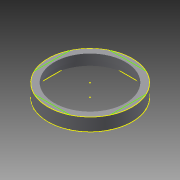
# Autodesk Inventor part: I53O
Saved by Autodesk Inventor 2014 (Build 180170000, 170)
## iProperties
Created: 2013-05-25
Part Number: I53O
Material: Generisch
Document SubType Name: Modeling
Designer: Felix
Density: 1 g/cm^3
Appearance: Vorgabe
Author: Felix
Autodesk Inventor part; units mm, degrees
ref_plane "YZ Plane" through (0, 0, 0) normal (1, 0, 0) x (0, 1, 0)
ref_plane "XZ Plane" through (0, 0, 0) normal (0, 1, 0) x (-1, 0, 0)
ref_plane "XY Plane" through (0, 0, 0) normal (0, 0, 1) x (1, 0, 0)
sketch "Sketch1" plane through (0, 0, 0) normal (0, 0, 1) x (1, 0, 0)
  circle A0 centre (0, 0) radius 13.0482
  spline S0 degree 3 poles (1.4215, 11.0572) (1.4473, 10.9809) (1.4859, 10.8664) (1.5292, 10.7112) (1.5586, 10.5939) (1.5843, 10.4759) (1.6059, 10.357) (1.6236, 10.2374) (1.631, 10.1572) (1.6346, 10.117) knots -0.096663 -0.096663 -0.096663 -0.096663 -0.072499 -0.060415 -0.048332 -0.036249 -0.024166 -0.012083 0 0 0 0 projected
  arc A1 (1.9905, 10.0531) -> (1.6346, 10.117) centre (0, 0) ccw projected
  spline S1 degree 3 poles (1.9905, 10.0531) (2.0079, 10.0894) (2.0426, 10.1621) (2.1009, 10.268) (2.1626, 10.3719) (2.2278, 10.4737) (2.2962, 10.5733) (2.3908, 10.7038) (2.4669, 10.7977) (2.5176, 10.8602) knots -0.096663 -0.096663 -0.096663 -0.096663 -0.084581 -0.072498 -0.060415 -0.048331 -0.036248 -0.024165 0 0 0 0 projected
  arc A2 (2.7193, 10.8115) -> (2.5176, 10.8602) centre (0, 0) ccw projected
  spline S2 degree 3 poles (2.7193, 10.8115) (2.7359, 10.7327) (2.7607, 10.6144) (2.7853, 10.4551) (2.8006, 10.3353) (2.8122, 10.215) (2.8196, 10.0943) (2.8231, 9.9735) (2.8208, 9.893) (2.8197, 9.8527) knots -0.096663 -0.096663 -0.096663 -0.096663 -0.072499 -0.060415 -0.048332 -0.036249 -0.024166 -0.012083 0 0 0 0 projected
  arc A3 (3.1655, 9.7471) -> (2.8197, 9.8527) centre (0, 0) ccw projected
  spline S3 degree 3 poles (3.1655, 9.7471) (3.1871, 9.7811) (3.2302, 9.8492) (3.3006, 9.9475) (3.3741, 10.0433) (3.4509, 10.1367) (3.5306, 10.2275) (3.64, 10.3459) (3.7266, 10.4301) (3.7844, 10.4863) knots -0.096663 -0.096663 -0.096663 -0.096663 -0.084581 -0.072498 -0.060415 -0.048331 -0.036248 -0.024165 0 0 0 0 projected
  arc A4 (3.9789, 10.414) -> (3.7844, 10.4863) centre (0, 0) ccw projected
  spline S4 degree 3 poles (3.9789, 10.414) (3.986, 10.3337) (3.9967, 10.2134) (4.0023, 10.0523) (4.0033, 9.9315) (4.0006, 9.8106) (3.9937, 9.69) (3.9828, 9.5696) (3.9711, 9.4899) (3.9652, 9.45) knots -0.096663 -0.096663 -0.096663 -0.096663 -0.072499 -0.060415 -0.048332 -0.036249 -0.024166 -0.012083 0 0 0 0 projected
  arc A5 (4.2961, 9.3043) -> (3.9652, 9.45) centre (0, 0) ccw projected
  spline S5 degree 3 poles (4.2961, 9.3043) (4.3215, 9.3355) (4.3724, 9.398) (4.4539, 9.4873) (4.5383, 9.5738) (4.6256, 9.6574) (4.7154, 9.7382) (4.838, 9.8428) (4.9341, 9.9161) (4.9981, 9.9651) knots -0.096663 -0.096663 -0.096663 -0.096663 -0.084581 -0.072498 -0.060415 -0.048331 -0.036248 -0.024165 0 0 0 0 projected
  arc A6 (5.1827, 9.8703) -> (4.9981, 9.9651) centre (0, 0) ccw projected
  spline S6 degree 3 poles (5.1827, 9.8703) (5.1803, 9.7898) (5.1766, 9.669) (5.1631, 9.5084) (5.1498, 9.3883) (5.1328, 9.2686) (5.1117, 9.1496) (5.0867, 9.0314) (5.0656, 8.9536) (5.0551, 8.9147) knots -0.096663 -0.096663 -0.096663 -0.096663 -0.072499 -0.060415 -0.048332 -0.036249 -0.024166 -0.012083 0 0 0 0 projected
  arc A7 (5.3664, 8.7309) -> (5.0551, 8.9147) centre (0, 0) ccw projected
  spline S7 degree 3 poles (5.3664, 8.7309) (5.3954, 8.7589) (5.4533, 8.8149) (5.5447, 8.8939) (5.6388, 8.9698) (5.7353, 9.0425) (5.8341, 9.1121) (5.9682, 9.2015) (6.0723, 9.263) (6.1416, 9.304) knots -0.096663 -0.096663 -0.096663 -0.096663 -0.084581 -0.072498 -0.060415 -0.048331 -0.036248 -0.024165 0 0 0 0 projected
  arc A8 (6.3137, 9.1881) -> (6.1416, 9.304) centre (0, 0) ccw projected
  spline S8 degree 3 poles (6.3137, 9.1881) (6.3018, 9.1084) (6.2839, 8.9889) (6.2515, 8.831) (6.2241, 8.7133) (6.193, 8.5965) (6.158, 8.4808) (6.1192, 8.3664) (6.089, 8.2916) (6.074, 8.2543) knots -0.096663 -0.096663 -0.096663 -0.096663 -0.072499 -0.060415 -0.048332 -0.036249 -0.024166 -0.012083 0 0 0 0 projected
  arc A9 (6.3614, 8.0349) -> (6.074, 8.2543) centre (0, 0) ccw projected
  spline S9 degree 3 poles (6.3614, 8.0349) (6.3934, 8.0593) (6.4576, 8.108) (6.5577, 8.1757) (6.6601, 8.24) (6.7646, 8.3007) (6.8709, 8.3581) (7.0146, 8.431) (7.1252, 8.4798) (7.1989, 8.5123) knots -0.096663 -0.096663 -0.096663 -0.096663 -0.084581 -0.072498 -0.060415 -0.048331 -0.036248 -0.024165 0 0 0 0 projected
  arc A10 (7.3561, 8.3768) -> (7.1989, 8.5123) centre (0, 0) ccw projected
  spline S10 degree 3 poles (7.3561, 8.3768) (7.3348, 8.2991) (7.3029, 8.1825) (7.2521, 8.0296) (7.2109, 7.916) (7.1663, 7.8037) (7.1179, 7.693) (7.0657, 7.5839) (7.027, 7.5133) (7.0076, 7.478) knots -0.096663 -0.096663 -0.096663 -0.096663 -0.072499 -0.060415 -0.048332 -0.036249 -0.024166 -0.012083 0 0 0 0 projected
  arc A11 (7.267, 7.2261) -> (7.0076, 7.478) centre (0, 0) ccw projected
  spline S11 degree 3 poles (7.267, 7.2261) (7.3017, 7.2465) (7.3712, 7.2874) (7.4787, 7.3427) (7.5879, 7.3944) (7.6988, 7.4424) (7.8112, 7.4868) (7.9625, 7.5422) (8.0781, 7.5775) (8.1552, 7.6011) knots -0.096663 -0.096663 -0.096663 -0.096663 -0.084581 -0.072498 -0.060415 -0.048331 -0.036248 -0.024165 0 0 0 0 projected
  arc A12 (8.2952, 7.448) -> (8.1552, 7.6011) centre (0, 0) ccw projected
  spline S12 degree 3 poles (8.2952, 7.448) (8.2649, 7.3734) (8.2194, 7.2614) (8.1509, 7.1155) (8.0966, 7.0076) (8.039, 6.9013) (7.9778, 6.7971) (7.9131, 6.695) (7.8663, 6.6294) (7.8429, 6.5967) knots -0.096663 -0.096663 -0.096663 -0.096663 -0.072499 -0.060415 -0.048332 -0.036249 -0.024166 -0.012083 0 0 0 0 projected
  arc A13 (8.0707, 6.3159) -> (7.8429, 6.5967) centre (0, 0) ccw projected
  spline S13 degree 3 poles (8.0707, 6.3159) (8.1076, 6.3321) (8.1814, 6.3644) (8.2946, 6.4066) (8.4092, 6.4451) (8.525, 6.4796) (8.6419, 6.5104) (8.7987, 6.5475) (8.9176, 6.5689) (8.9969, 6.5832) knots -0.096663 -0.096663 -0.096663 -0.096663 -0.084581 -0.072498 -0.060415 -0.048331 -0.036248 -0.024165 0 0 0 0 projected
  arc A14 (9.1179, 6.4146) -> (8.9969, 6.5832) centre (0, 0) ccw projected
  spline S14 degree 3 poles (9.1179, 6.4146) (9.079, 6.3441) (9.0206, 6.2383) (8.9352, 6.1016) (8.8686, 6.0008) (8.7988, 5.9021) (8.7257, 5.8059) (8.6494, 5.7121) (8.5952, 5.6525) (8.568, 5.6228) knots -0.096663 -0.096663 -0.096663 -0.096663 -0.072499 -0.060415 -0.048332 -0.036249 -0.024166 -0.012083 0 0 0 0 projected
  arc A15 (8.761, 5.317) -> (8.568, 5.6228) centre (0, 0) ccw projected
  spline S15 degree 3 poles (8.761, 5.317) (8.7996, 5.3287) (8.8767, 5.3521) (8.9941, 5.3806) (9.1125, 5.4052) (9.2316, 5.4258) (9.3512, 5.4426) (9.5113, 5.4609) (9.632, 5.4681) (9.7124, 5.4729) knots -0.096663 -0.096663 -0.096663 -0.096663 -0.084581 -0.072498 -0.060415 -0.048331 -0.036248 -0.024165 0 0 0 0 projected
  arc A16 (9.8126, 5.2912) -> (9.7124, 5.4729) centre (0, 0) ccw projected
  spline S16 degree 3 poles (9.8126, 5.2912) (9.7656, 5.2258) (9.6951, 5.1276) (9.5942, 5.002) (9.516, 4.9097) (9.4351, 4.82) (9.3511, 4.7331) (9.2643, 4.649) (9.2034, 4.5963) (9.1729, 4.5699) knots -0.096663 -0.096663 -0.096663 -0.096663 -0.072499 -0.060415 -0.048332 -0.036249 -0.024166 -0.012083 0 0 0 0 projected
  arc A17 (9.3284, 4.2435) -> (9.1729, 4.5699) centre (0, 0) ccw projected
  spline S17 degree 3 poles (9.3284, 4.2435) (9.3681, 4.2506) (9.4474, 4.2647) (9.5674, 4.2791) (9.6878, 4.2896) (9.8085, 4.2959) (9.9293, 4.2984) (10.0904, 4.2976) (10.2111, 4.2905) (10.2915, 4.2858) knots -0.096663 -0.096663 -0.096663 -0.096663 -0.084581 -0.072498 -0.060415 -0.048331 -0.036248 -0.024165 0 0 0 0 projected
  arc A18 (10.3695, 4.0935) -> (10.2915, 4.2858) centre (0, 0) ccw projected
  spline S18 degree 3 poles (10.3695, 4.0935) (10.3151, 4.0341) (10.2335, 3.9449) (10.1184, 3.8321) (10.0299, 3.7498) (9.939, 3.6703) (9.8453, 3.5939) (9.7491, 3.5206) (9.6824, 3.4755) (9.649, 3.4529) knots -0.096663 -0.096663 -0.096663 -0.096663 -0.072499 -0.060415 -0.048332 -0.036249 -0.024166 -0.012083 0 0 0 0 projected
  arc A19 (9.7648, 3.1104) -> (9.649, 3.4529) centre (0, 0) ccw projected
  spline S19 degree 3 poles (9.7648, 3.1104) (9.805, 3.1127) (9.8855, 3.1174) (10.0063, 3.1175) (10.1271, 3.1136) (10.2477, 3.1056) (10.368, 3.0939) (10.5279, 3.074) (10.6469, 3.0527) (10.7262, 3.0385) knots -0.096663 -0.096663 -0.096663 -0.096663 -0.084581 -0.072498 -0.060415 -0.048331 -0.036248 -0.024165 0 0 0 0 projected
  arc A20 (10.7809, 2.8383) -> (10.7262, 3.0385) centre (0, 0) ccw projected
  spline S20 degree 3 poles (10.7809, 2.8383) (10.7198, 2.7858) (10.6282, 2.7069) (10.5006, 2.6085) (10.403, 2.5372) (10.3033, 2.469) (10.2013, 2.4042) (10.0971, 2.3429) (10.0255, 2.306) (9.9897, 2.2875) knots -0.096663 -0.096663 -0.096663 -0.096663 -0.072499 -0.060415 -0.048332 -0.036249 -0.024166 -0.012083 0 0 0 0 projected
  arc A21 (10.0642, 1.9337) -> (9.9897, 2.2875) centre (0, 0) ccw projected
  spline S21 degree 3 poles (10.0642, 1.9337) (10.1044, 1.9312) (10.1848, 1.9263) (10.3048, 1.9121) (10.4243, 1.894) (10.5431, 1.8718) (10.6611, 1.8459) (10.8176, 1.8073) (10.9332, 1.772) (11.0103, 1.7485) knots -0.096663 -0.096663 -0.096663 -0.096663 -0.084581 -0.072498 -0.060415 -0.048331 -0.036248 -0.024165 0 0 0 0 projected
  arc A22 (11.0409, 1.5433) -> (11.0103, 1.7485) centre (0, 0) ccw projected
  spline S22 degree 3 poles (11.0409, 1.5433) (10.9741, 1.4983) (10.8738, 1.4309) (10.7354, 1.3482) (10.6301, 1.289) (10.523, 1.2331) (10.414, 1.1808) (10.3033, 1.1322) (10.2279, 1.104) (10.1901, 1.0899) knots -0.096663 -0.096663 -0.096663 -0.096663 -0.072499 -0.060415 -0.048332 -0.036249 -0.024166 -0.012083 0 0 0 0 projected
  arc A23 (10.2222, 0.7298) -> (10.1901, 1.0899) centre (0, 0) ccw projected
  spline S23 degree 3 poles (10.2222, 0.7298) (10.2619, 0.7226) (10.3411, 0.7082) (10.4587, 0.6799) (10.5752, 0.6478) (10.6905, 0.6117) (10.8046, 0.572) (10.9554, 0.5152) (11.066, 0.4665) (11.1398, 0.434) knots -0.096663 -0.096663 -0.096663 -0.096663 -0.084581 -0.072498 -0.060415 -0.048331 -0.036248 -0.024165 0 0 0 0 projected
  arc A24 (11.1459, 0.2266) -> (11.1398, 0.434) centre (0, 0) ccw projected
  spline S24 degree 3 poles (11.1459, 0.2266) (11.0742, 0.1899) (10.9667, 0.1348) (10.8196, 0.069) (10.708, 0.0227) (10.595, -0.0202) (10.4806, -0.0592) (10.3649, -0.0943) (10.2866, -0.1134) (10.2475, -0.1229) knots -0.096663 -0.096663 -0.096663 -0.096663 -0.072499 -0.060415 -0.048332 -0.036249 -0.024166 -0.012083 0 0 0 0 projected
  arc A25 (10.2368, -0.4843) -> (10.2475, -0.1229) centre (0, 0) ccw projected
  spline S25 degree 3 poles (10.2368, -0.4843) (10.2753, -0.4962) (10.3523, -0.5199) (10.4657, -0.5618) (10.5775, -0.6075) (10.6878, -0.657) (10.7965, -0.7099) (10.9394, -0.7842) (11.0435, -0.8456) (11.1129, -0.8865) knots -0.096663 -0.096663 -0.096663 -0.096663 -0.084581 -0.072498 -0.060415 -0.048331 -0.036248 -0.024165 0 0 0 0 projected
  arc A26 (11.0945, -1.0932) -> (11.1129, -0.8865) centre (0, 0) ccw projected
  spline S26 degree 3 poles (11.0945, -1.0932) (11.019, -1.1212) (10.9057, -1.1633) (10.7518, -1.2111) (10.6355, -1.2439) (10.5182, -1.2731) (10.4, -1.2983) (10.281, -1.3196) (10.201, -1.3292) (10.161, -1.3341) knots -0.096663 -0.096663 -0.096663 -0.096663 -0.072499 -0.060415 -0.048332 -0.036249 -0.024166 -0.012083 0 0 0 0 projected
  arc A27 (10.1077, -1.6917) -> (10.161, -1.3341) centre (0, 0) ccw projected
  spline S27 degree 3 poles (10.1077, -1.6917) (10.1445, -1.708) (10.2182, -1.7406) (10.3258, -1.7957) (10.4315, -1.8543) (10.5351, -1.9165) (10.6367, -1.9818) (10.7699, -2.0725) (10.866, -2.1458) (10.9301, -2.1947) knots -0.096663 -0.096663 -0.096663 -0.096663 -0.084581 -0.072498 -0.060415 -0.048331 -0.036248 -0.024165 0 0 0 0 projected
  arc A28 (10.8873, -2.3977) -> (10.9301, -2.1947) centre (0, 0) ccw projected
  spline S28 degree 3 poles (10.8873, -2.3977) (10.809, -2.4166) (10.6915, -2.4449) (10.5331, -2.4742) (10.4137, -2.4931) (10.2938, -2.5082) (10.1735, -2.5192) (10.0528, -2.5263) (9.9722, -2.5264) (9.9319, -2.5265) knots -0.096663 -0.096663 -0.096663 -0.096663 -0.072499 -0.060415 -0.048332 -0.036249 -0.024166 -0.012083 0 0 0 0 projected
  arc A29 (9.8366, -2.8753) -> (9.9319, -2.5265) centre (0, 0) ccw projected
  spline S29 degree 3 poles (9.8366, -2.8753) (9.8713, -2.8958) (9.9406, -2.9369) (10.0409, -3.0043) (10.1389, -3.075) (10.2345, -3.149) (10.3277, -3.226) (10.4492, -3.3318) (10.536, -3.4159) (10.5938, -3.472) knots -0.096663 -0.096663 -0.096663 -0.096663 -0.084581 -0.072498 -0.060415 -0.048331 -0.036248 -0.024165 0 0 0 0 projected
  arc A30 (10.5273, -3.6686) -> (10.5938, -3.472) centre (0, 0) ccw projected
  spline S30 degree 3 poles (10.5273, -3.6686) (10.4473, -3.6781) (10.3273, -3.6923) (10.1665, -3.7027) (10.0457, -3.7073) (9.9249, -3.7081) (9.8041, -3.7048) (9.6834, -3.6975) (9.6034, -3.6881) (9.5634, -3.6834) knots -0.096663 -0.096663 -0.096663 -0.096663 -0.072499 -0.060415 -0.048332 -0.036249 -0.024166 -0.012083 0 0 0 0 projected
  arc A31 (9.4275, -4.0185) -> (9.5634, -3.6834) centre (0, 0) ccw projected
  spline S31 degree 3 poles (9.4275, -4.0185) (9.4595, -4.043) (9.5234, -4.092) (9.6151, -4.1708) (9.7041, -4.2526) (9.7902, -4.3374) (9.8736, -4.4248) (9.9818, -4.5442) (10.058, -4.6381) (10.1088, -4.7006) knots -0.096663 -0.096663 -0.096663 -0.096663 -0.084581 -0.072498 -0.060415 -0.048331 -0.036248 -0.024165 0 0 0 0 projected
  arc A32 (10.0196, -4.8879) -> (10.1088, -4.7006) centre (0, 0) ccw projected
  spline S32 degree 3 poles (10.0196, -4.8879) (9.939, -4.8879) (9.8181, -4.8878) (9.6572, -4.8791) (9.5368, -4.8694) (9.4167, -4.8559) (9.2971, -4.8384) (9.1781, -4.8168) (9.0998, -4.7981) (9.0606, -4.7887) knots -0.096663 -0.096663 -0.096663 -0.096663 -0.072499 -0.060415 -0.048332 -0.036249 -0.024166 -0.012083 0 0 0 0 projected
  arc A33 (8.8861, -5.1053) -> (9.0606, -4.7887) centre (0, 0) ccw projected
  spline S33 degree 3 poles (8.8861, -5.1053) (8.9149, -5.1334) (8.9726, -5.1897) (9.0543, -5.2788) (9.133, -5.3705) (9.2085, -5.4649) (9.281, -5.5615) (9.3743, -5.6929) (9.4388, -5.7951) (9.4819, -5.8632) knots -0.096663 -0.096663 -0.096663 -0.096663 -0.084581 -0.072498 -0.060415 -0.048331 -0.036248 -0.024165 0 0 0 0 projected
  arc A34 (9.3711, -6.0387) -> (9.4819, -5.8632) centre (0, 0) ccw projected
  spline S34 degree 3 poles (9.3711, -6.0387) (9.2911, -6.0291) (9.1711, -6.0147) (9.0124, -5.987) (8.8939, -5.9631) (8.7762, -5.9356) (8.6596, -5.904) (8.544, -5.8686) (8.4684, -5.8407) (8.4307, -5.8267) knots -0.096663 -0.096663 -0.096663 -0.096663 -0.072499 -0.060415 -0.048332 -0.036249 -0.024166 -0.012083 0 0 0 0 projected
  arc A35 (8.2199, -6.1205) -> (8.4307, -5.8267) centre (0, 0) ccw projected
  spline S35 degree 3 poles (8.2199, -6.1205) (8.2452, -6.1518) (8.2958, -6.2144) (8.3664, -6.3126) (8.4337, -6.413) (8.4975, -6.5156) (8.5581, -6.6202) (8.6352, -6.7617) (8.6872, -6.8708) (8.7219, -6.9435) knots -0.096663 -0.096663 -0.096663 -0.096663 -0.084581 -0.072498 -0.060415 -0.048331 -0.036248 -0.024165 0 0 0 0 projected
  arc A36 (8.5911, -7.1046) -> (8.7219, -6.9435) centre (0, 0) ccw projected
  spline S36 degree 3 poles (8.5911, -7.1046) (8.5128, -7.0857) (8.3954, -7.0572) (8.241, -7.0109) (8.1262, -6.9732) (8.0126, -6.9319) (7.9005, -6.8868) (7.79, -6.8379) (7.7182, -6.8013) (7.6823, -6.7829) knots -0.096663 -0.096663 -0.096663 -0.096663 -0.072499 -0.060415 -0.048332 -0.036249 -0.024166 -0.012083 0 0 0 0 projected
  arc A37 (7.4383, -7.0497) -> (7.6823, -6.7829) centre (0, 0) ccw projected
  spline S37 degree 3 poles (7.4383, -7.0497) (7.4597, -7.0838) (7.5026, -7.152) (7.5611, -7.2578) (7.616, -7.3654) (7.6672, -7.4749) (7.715, -7.5859) (7.7748, -7.7355) (7.8136, -7.85) (7.8394, -7.9263) knots -0.096663 -0.096663 -0.096663 -0.096663 -0.084581 -0.072498 -0.060415 -0.048331 -0.036248 -0.024165 0 0 0 0 projected
  arc A38 (7.6905, -8.0709) -> (7.8394, -7.9263) centre (0, 0) ccw projected
  spline S38 degree 3 poles (7.6905, -8.0709) (7.615, -8.0428) (7.5018, -8.0006) (7.354, -7.9364) (7.2444, -7.8854) (7.1365, -7.8309) (7.0306, -7.7728) (6.9265, -7.7113) (6.8596, -7.6664) (6.8262, -7.6439) knots -0.096663 -0.096663 -0.096663 -0.096663 -0.072499 -0.060415 -0.048332 -0.036249 -0.024166 -0.012083 0 0 0 0 projected
  arc A39 (6.5523, -7.88) -> (6.8262, -7.6439) centre (0, 0) ccw projected
  spline S39 degree 3 poles (6.5523, -7.88) (6.5696, -7.9164) (6.6041, -7.9892) (6.6496, -8.1011) (6.6914, -8.2145) (6.7293, -8.3293) (6.7637, -8.4451) (6.8053, -8.6008) (6.8303, -8.7191) (6.8469, -8.7979) knots -0.096663 -0.096663 -0.096663 -0.096663 -0.084581 -0.072498 -0.060415 -0.048331 -0.036248 -0.024165 0 0 0 0 projected
  arc A40 (6.682, -8.9238) -> (6.8469, -8.7979) centre (0, 0) ccw projected
  spline S40 degree 3 poles (6.682, -8.9238) (6.6103, -8.887) (6.5028, -8.8317) (6.3637, -8.7505) (6.261, -8.6868) (6.1602, -8.62) (6.0619, -8.5498) (5.9659, -8.4764) (5.9048, -8.4239) (5.8742, -8.3976) knots -0.096663 -0.096663 -0.096663 -0.096663 -0.072499 -0.060415 -0.048332 -0.036249 -0.024166 -0.012083 0 0 0 0 projected
  arc A41 (5.5743, -8.5996) -> (5.8742, -8.3976) centre (0, 0) ccw projected
  spline S41 degree 3 poles (5.5743, -8.5996) (5.5871, -8.6378) (5.6128, -8.7142) (5.6448, -8.8307) (5.6729, -8.9483) (5.697, -9.0667) (5.7173, -9.1858) (5.7403, -9.3453) (5.7511, -9.4657) (5.7583, -9.5459) knots -0.096663 -0.096663 -0.096663 -0.096663 -0.084581 -0.072498 -0.060415 -0.048331 -0.036248 -0.024165 0 0 0 0 projected
  arc A42 (5.5797, -9.6515) -> (5.7583, -9.5459) centre (0, 0) ccw projected
  spline S42 degree 3 poles (5.5797, -9.6515) (5.5128, -9.6064) (5.4126, -9.5389) (5.2841, -9.4417) (5.1896, -9.3664) (5.0975, -9.2881) (5.0081, -9.2068) (4.9215, -9.1225) (4.867, -9.0631) (4.8397, -9.0335) knots -0.096663 -0.096663 -0.096663 -0.096663 -0.072499 -0.060415 -0.048332 -0.036249 -0.024166 -0.012083 0 0 0 0 projected
  arc A43 (4.5181, -9.1985) -> (4.8397, -9.0335) centre (0, 0) ccw projected
  spline S43 degree 3 poles (4.5181, -9.1985) (4.5263, -9.238) (4.5428, -9.3169) (4.5607, -9.4364) (4.5747, -9.5564) (4.5846, -9.6769) (4.5908, -9.7976) (4.5947, -9.9587) (4.5912, -10.0795) (4.5889, -10.16) knots -0.096663 -0.096663 -0.096663 -0.096663 -0.084581 -0.072498 -0.060415 -0.048331 -0.036248 -0.024165 0 0 0 0 projected
  arc A44 (4.399, -10.2436) -> (4.5889, -10.16) centre (0, 0) ccw projected
  spline S44 degree 3 poles (4.399, -10.2436) (4.338, -10.191) (4.2465, -10.1121) (4.1303, -10.0004) (4.0454, -9.9144) (3.9632, -9.8258) (3.8841, -9.7345) (3.808, -9.6405) (3.7609, -9.5751) (3.7374, -9.5425) knots -0.096663 -0.096663 -0.096663 -0.096663 -0.072499 -0.060415 -0.048332 -0.036249 -0.024166 -0.012083 0 0 0 0 projected
  arc A45 (3.3984, -9.6684) -> (3.7374, -9.5425) centre (0, 0) ccw projected
  spline S45 degree 3 poles (3.3984, -9.6684) (3.4019, -9.7085) (3.4089, -9.7887) (3.4127, -9.9096) (3.4124, -10.0304) (3.4079, -10.1512) (3.3998, -10.2718) (3.3846, -10.4322) (3.3669, -10.5517) (3.355, -10.6314) knots -0.096663 -0.096663 -0.096663 -0.096663 -0.084581 -0.072498 -0.060415 -0.048331 -0.036248 -0.024165 0 0 0 0 projected
  arc A46 (3.1566, -10.692) -> (3.355, -10.6314) centre (0, 0) ccw projected
  spline S46 degree 3 poles (3.1566, -10.692) (3.1022, -10.6326) (3.0207, -10.5433) (2.9185, -10.4187) (2.8444, -10.3233) (2.7732, -10.2256) (2.7055, -10.1255) (2.6411, -10.0232) (2.602, -9.9528) (2.5825, -9.9175) knots -0.096663 -0.096663 -0.096663 -0.096663 -0.072499 -0.060415 -0.048332 -0.036249 -0.024166 -0.012083 0 0 0 0 projected
  arc A47 (2.2311, -10.0024) -> (2.5825, -9.9175) centre (0, 0) ccw projected
  spline S47 degree 3 poles (2.2311, -10.0024) (2.2298, -10.0427) (2.2273, -10.1232) (2.2167, -10.2436) (2.2021, -10.3636) (2.1834, -10.483) (2.161, -10.6018) (2.127, -10.7593) (2.0952, -10.8759) (2.074, -10.9536) knots -0.096663 -0.096663 -0.096663 -0.096663 -0.084581 -0.072498 -0.060415 -0.048331 -0.036248 -0.024165 0 0 0 0 projected
  arc A48 (1.8698, -10.9903) -> (2.074, -10.9536) centre (0, 0) ccw projected
  spline S48 degree 3 poles (1.8698, -10.9903) (1.8229, -10.9248) (1.7525, -10.8266) (1.6658, -10.6908) (1.6034, -10.5872) (1.5443, -10.4818) (1.4889, -10.3744) (1.437, -10.2652) (1.4066, -10.1906) (1.3914, -10.1533) knots -0.096663 -0.096663 -0.096663 -0.096663 -0.072499 -0.060415 -0.048332 -0.036249 -0.024166 -0.012083 0 0 0 0 projected
  arc A49 (1.0324, -10.1961) -> (1.3914, -10.1533) centre (0, 0) ccw projected
  spline S49 degree 3 poles (1.0324, -10.1961) (1.0264, -10.2359) (1.0143, -10.3156) (0.9896, -10.4339) (0.9609, -10.5513) (0.9282, -10.6677) (0.892, -10.7829) (0.8396, -10.9353) (0.7942, -11.0474) (0.764, -11.122) knots -0.096663 -0.096663 -0.096663 -0.096663 -0.084581 -0.072498 -0.060415 -0.048331 -0.036248 -0.024165 0 0 0 0 projected
  arc A50 (0.5568, -11.1343) -> (0.764, -11.122) centre (0, 0) ccw projected
  spline S50 degree 3 poles (0.5568, -11.1343) (0.518, -11.0637) (0.4597, -10.9579) (0.3896, -10.8128) (0.34, -10.7026) (0.2938, -10.5909) (0.2514, -10.4777) (0.2129, -10.3632) (0.1915, -10.2855) (0.1808, -10.2466) knots -0.096663 -0.096663 -0.096663 -0.096663 -0.072499 -0.060415 -0.048332 -0.036249 -0.024166 -0.012083 0 0 0 0 projected
  arc A51 (-0.1808, -10.2466) -> (0.1808, -10.2466) centre (0, 0) ccw projected
  spline S51 degree 3 poles (-0.1808, -10.2466) (-0.1915, -10.2855) (-0.2129, -10.3632) (-0.2514, -10.4777) (-0.2938, -10.5909) (-0.34, -10.7026) (-0.3896, -10.8128) (-0.4597, -10.9579) (-0.518, -11.0637) (-0.5568, -11.1343) knots -0.096663 -0.096663 -0.096663 -0.096663 -0.084581 -0.072498 -0.060415 -0.048331 -0.036248 -0.024165 0 0 0 0 projected
  arc A52 (-0.764, -11.122) -> (-0.5568, -11.1343) centre (0, 0) ccw projected
  spline S52 degree 3 poles (-0.764, -11.122) (-0.7942, -11.0474) (-0.8396, -10.9353) (-0.892, -10.7829) (-0.9282, -10.6677) (-0.9609, -10.5513) (-0.9896, -10.4339) (-1.0143, -10.3156) (-1.0264, -10.2359) (-1.0324, -10.1961) knots -0.096663 -0.096663 -0.096663 -0.096663 -0.072499 -0.060415 -0.048332 -0.036249 -0.024166 -0.012083 0 0 0 0 projected
  arc A53 (-1.3914, -10.1533) -> (-1.0324, -10.1961) centre (0, 0) ccw projected
  spline S53 degree 3 poles (-1.3914, -10.1533) (-1.4066, -10.1906) (-1.437, -10.2652) (-1.4889, -10.3744) (-1.5443, -10.4818) (-1.6034, -10.5872) (-1.6658, -10.6908) (-1.7525, -10.8266) (-1.8229, -10.9248) (-1.8698, -10.9903) knots -0.096663 -0.096663 -0.096663 -0.096663 -0.084581 -0.072498 -0.060415 -0.048331 -0.036248 -0.024165 0 0 0 0 projected
  arc A54 (-2.074, -10.9536) -> (-1.8698, -10.9903) centre (0, 0) ccw projected
  spline S54 degree 3 poles (-2.074, -10.9536) (-2.0952, -10.8759) (-2.127, -10.7593) (-2.161, -10.6018) (-2.1834, -10.483) (-2.2021, -10.3636) (-2.2167, -10.2436) (-2.2273, -10.1232) (-2.2298, -10.0427) (-2.2311, -10.0024) knots -0.096663 -0.096663 -0.096663 -0.096663 -0.072499 -0.060415 -0.048332 -0.036249 -0.024166 -0.012083 0 0 0 0 projected
  arc A55 (-2.5825, -9.9175) -> (-2.2311, -10.0024) centre (0, 0) ccw projected
  spline S55 degree 3 poles (-2.5825, -9.9175) (-2.602, -9.9528) (-2.6411, -10.0232) (-2.7055, -10.1255) (-2.7732, -10.2256) (-2.8444, -10.3233) (-2.9185, -10.4187) (-3.0207, -10.5433) (-3.1022, -10.6326) (-3.1566, -10.692) knots -0.096663 -0.096663 -0.096663 -0.096663 -0.084581 -0.072498 -0.060415 -0.048331 -0.036248 -0.024165 0 0 0 0 projected
  arc A56 (-3.355, -10.6314) -> (-3.1566, -10.692) centre (0, 0) ccw projected
  spline S56 degree 3 poles (-3.355, -10.6314) (-3.3669, -10.5517) (-3.3846, -10.4322) (-3.3998, -10.2718) (-3.4079, -10.1512) (-3.4124, -10.0304) (-3.4127, -9.9096) (-3.4089, -9.7887) (-3.4019, -9.7085) (-3.3984, -9.6684) knots -0.096663 -0.096663 -0.096663 -0.096663 -0.072499 -0.060415 -0.048332 -0.036249 -0.024166 -0.012083 0 0 0 0 projected
  arc A57 (-3.7374, -9.5425) -> (-3.3984, -9.6684) centre (0, 0) ccw projected
  spline S57 degree 3 poles (-3.7374, -9.5425) (-3.7609, -9.5751) (-3.808, -9.6405) (-3.8841, -9.7345) (-3.9632, -9.8258) (-4.0454, -9.9144) (-4.1303, -10.0004) (-4.2465, -10.1121) (-4.338, -10.191) (-4.399, -10.2436) knots -0.096663 -0.096663 -0.096663 -0.096663 -0.084581 -0.072498 -0.060415 -0.048331 -0.036248 -0.024165 0 0 0 0 projected
  arc A58 (-4.5889, -10.16) -> (-4.399, -10.2436) centre (0, 0) ccw projected
  spline S58 degree 3 poles (-4.5889, -10.16) (-4.5912, -10.0795) (-4.5947, -9.9587) (-4.5908, -9.7976) (-4.5846, -9.6769) (-4.5747, -9.5564) (-4.5607, -9.4364) (-4.5428, -9.3169) (-4.5263, -9.238) (-4.5181, -9.1985) knots -0.096663 -0.096663 -0.096663 -0.096663 -0.072499 -0.060415 -0.048332 -0.036249 -0.024166 -0.012083 0 0 0 0 projected
  arc A59 (-4.8397, -9.0335) -> (-4.5181, -9.1985) centre (0, 0) ccw projected
  spline S59 degree 3 poles (-4.8397, -9.0335) (-4.867, -9.0631) (-4.9215, -9.1225) (-5.0081, -9.2068) (-5.0975, -9.2881) (-5.1896, -9.3664) (-5.2841, -9.4417) (-5.4126, -9.5389) (-5.5128, -9.6064) (-5.5797, -9.6515) knots -0.096663 -0.096663 -0.096663 -0.096663 -0.084581 -0.072498 -0.060415 -0.048331 -0.036248 -0.024165 0 0 0 0 projected
  arc A60 (-5.7583, -9.5459) -> (-5.5797, -9.6515) centre (0, 0) ccw projected
  spline S60 degree 3 poles (-5.7583, -9.5459) (-5.7511, -9.4657) (-5.7403, -9.3453) (-5.7173, -9.1858) (-5.697, -9.0667) (-5.6729, -8.9483) (-5.6448, -8.8307) (-5.6128, -8.7142) (-5.5871, -8.6378) (-5.5743, -8.5996) knots -0.096663 -0.096663 -0.096663 -0.096663 -0.072499 -0.060415 -0.048332 -0.036249 -0.024166 -0.012083 0 0 0 0 projected
  arc A61 (-5.8742, -8.3976) -> (-5.5743, -8.5996) centre (0, 0) ccw projected
  spline S61 degree 3 poles (-5.8742, -8.3976) (-5.9048, -8.4239) (-5.9659, -8.4764) (-6.0619, -8.5498) (-6.1602, -8.62) (-6.261, -8.6868) (-6.3637, -8.7505) (-6.5028, -8.8317) (-6.6103, -8.887) (-6.682, -8.9238) knots -0.096663 -0.096663 -0.096663 -0.096663 -0.084581 -0.072498 -0.060415 -0.048331 -0.036248 -0.024165 0 0 0 0 projected
  arc A62 (-6.8469, -8.7979) -> (-6.682, -8.9238) centre (0, 0) ccw projected
  spline S62 degree 3 poles (-6.8469, -8.7979) (-6.8303, -8.7191) (-6.8053, -8.6008) (-6.7637, -8.4451) (-6.7293, -8.3293) (-6.6914, -8.2145) (-6.6496, -8.1011) (-6.6041, -7.9892) (-6.5696, -7.9164) (-6.5523, -7.88) knots -0.096663 -0.096663 -0.096663 -0.096663 -0.072499 -0.060415 -0.048332 -0.036249 -0.024166 -0.012083 0 0 0 0 projected
  arc A63 (-6.8262, -7.6439) -> (-6.5523, -7.88) centre (0, 0) ccw projected
  spline S63 degree 3 poles (-6.8262, -7.6439) (-6.8596, -7.6664) (-6.9265, -7.7113) (-7.0306, -7.7728) (-7.1365, -7.8309) (-7.2444, -7.8854) (-7.354, -7.9364) (-7.5018, -8.0006) (-7.615, -8.0428) (-7.6905, -8.0709) knots -0.096663 -0.096663 -0.096663 -0.096663 -0.084581 -0.072498 -0.060415 -0.048331 -0.036248 -0.024165 0 0 0 0 projected
  arc A64 (-7.8394, -7.9263) -> (-7.6905, -8.0709) centre (0, 0) ccw projected
  spline S64 degree 3 poles (-7.8394, -7.9263) (-7.8136, -7.85) (-7.7748, -7.7355) (-7.715, -7.5859) (-7.6672, -7.4749) (-7.616, -7.3654) (-7.5611, -7.2578) (-7.5026, -7.152) (-7.4597, -7.0838) (-7.4383, -7.0497) knots -0.096663 -0.096663 -0.096663 -0.096663 -0.072499 -0.060415 -0.048332 -0.036249 -0.024166 -0.012083 0 0 0 0 projected
  arc A65 (-7.6823, -6.7829) -> (-7.4383, -7.0497) centre (0, 0) ccw projected
  spline S65 degree 3 poles (-7.6823, -6.7829) (-7.7182, -6.8013) (-7.79, -6.8379) (-7.9005, -6.8868) (-8.0126, -6.9319) (-8.1262, -6.9732) (-8.241, -7.0109) (-8.3954, -7.0572) (-8.5128, -7.0857) (-8.5911, -7.1046) knots -0.096663 -0.096663 -0.096663 -0.096663 -0.084581 -0.072498 -0.060415 -0.048331 -0.036248 -0.024165 0 0 0 0 projected
  arc A66 (-8.7219, -6.9435) -> (-8.5911, -7.1046) centre (0, 0) ccw projected
  spline S66 degree 3 poles (-8.7219, -6.9435) (-8.6872, -6.8708) (-8.6352, -6.7617) (-8.5581, -6.6202) (-8.4975, -6.5156) (-8.4337, -6.413) (-8.3664, -6.3126) (-8.2958, -6.2144) (-8.2452, -6.1518) (-8.2199, -6.1205) knots -0.096663 -0.096663 -0.096663 -0.096663 -0.072499 -0.060415 -0.048332 -0.036249 -0.024166 -0.012083 0 0 0 0 projected
  arc A67 (-8.4307, -5.8267) -> (-8.2199, -6.1205) centre (0, 0) ccw projected
  spline S67 degree 3 poles (-8.4307, -5.8267) (-8.4684, -5.8407) (-8.544, -5.8686) (-8.6596, -5.904) (-8.7762, -5.9356) (-8.8939, -5.9631) (-9.0124, -5.987) (-9.1711, -6.0147) (-9.2911, -6.0291) (-9.3711, -6.0387) knots -0.096663 -0.096663 -0.096663 -0.096663 -0.084581 -0.072498 -0.060415 -0.048331 -0.036248 -0.024165 0 0 0 0 projected
  arc A68 (-9.4819, -5.8632) -> (-9.3711, -6.0387) centre (0, 0) ccw projected
  spline S68 degree 3 poles (-9.4819, -5.8632) (-9.4388, -5.7951) (-9.3743, -5.6929) (-9.281, -5.5615) (-9.2085, -5.4649) (-9.133, -5.3705) (-9.0543, -5.2788) (-8.9726, -5.1897) (-8.9149, -5.1334) (-8.8861, -5.1053) knots -0.096663 -0.096663 -0.096663 -0.096663 -0.072499 -0.060415 -0.048332 -0.036249 -0.024166 -0.012083 0 0 0 0 projected
  arc A69 (-9.0606, -4.7887) -> (-8.8861, -5.1053) centre (0, 0) ccw projected
  spline S69 degree 3 poles (-9.0606, -4.7887) (-9.0998, -4.7981) (-9.1781, -4.8168) (-9.2971, -4.8384) (-9.4167, -4.8559) (-9.5368, -4.8694) (-9.6572, -4.8791) (-9.8181, -4.8878) (-9.939, -4.8879) (-10.0196, -4.8879) knots -0.096663 -0.096663 -0.096663 -0.096663 -0.084581 -0.072498 -0.060415 -0.048331 -0.036248 -0.024165 0 0 0 0 projected
  arc A70 (-10.1088, -4.7006) -> (-10.0196, -4.8879) centre (0, 0) ccw projected
  spline S70 degree 3 poles (-10.1088, -4.7006) (-10.058, -4.6381) (-9.9818, -4.5442) (-9.8736, -4.4248) (-9.7902, -4.3374) (-9.7041, -4.2526) (-9.6151, -4.1708) (-9.5234, -4.092) (-9.4595, -4.043) (-9.4275, -4.0185) knots -0.096663 -0.096663 -0.096663 -0.096663 -0.072499 -0.060415 -0.048332 -0.036249 -0.024166 -0.012083 0 0 0 0 projected
  arc A71 (-9.5634, -3.6834) -> (-9.4275, -4.0185) centre (0, 0) ccw projected
  spline S71 degree 3 poles (-9.5634, -3.6834) (-9.6034, -3.6881) (-9.6834, -3.6975) (-9.8041, -3.7048) (-9.9249, -3.7081) (-10.0457, -3.7073) (-10.1665, -3.7027) (-10.3273, -3.6923) (-10.4473, -3.6781) (-10.5273, -3.6686) knots -0.096663 -0.096663 -0.096663 -0.096663 -0.084581 -0.072498 -0.060415 -0.048331 -0.036248 -0.024165 0 0 0 0 projected
  arc A72 (-10.5938, -3.472) -> (-10.5273, -3.6686) centre (0, 0) ccw projected
  spline S72 degree 3 poles (-10.5938, -3.472) (-10.536, -3.4159) (-10.4492, -3.3318) (-10.3277, -3.226) (-10.2345, -3.149) (-10.1389, -3.075) (-10.0409, -3.0043) (-9.9406, -2.9369) (-9.8713, -2.8958) (-9.8366, -2.8753) knots -0.096663 -0.096663 -0.096663 -0.096663 -0.072499 -0.060415 -0.048332 -0.036249 -0.024166 -0.012083 0 0 0 0 projected
  arc A73 (-9.9319, -2.5265) -> (-9.8366, -2.8753) centre (0, 0) ccw projected
  spline S73 degree 3 poles (-9.9319, -2.5265) (-9.9722, -2.5264) (-10.0528, -2.5263) (-10.1735, -2.5192) (-10.2938, -2.5082) (-10.4137, -2.4931) (-10.5331, -2.4742) (-10.6915, -2.4449) (-10.809, -2.4166) (-10.8873, -2.3977) knots -0.096663 -0.096663 -0.096663 -0.096663 -0.084581 -0.072498 -0.060415 -0.048331 -0.036248 -0.024165 0 0 0 0 projected
  arc A74 (-10.9301, -2.1947) -> (-10.8873, -2.3977) centre (0, 0) ccw projected
  spline S74 degree 3 poles (-10.9301, -2.1947) (-10.866, -2.1458) (-10.7699, -2.0725) (-10.6367, -1.9818) (-10.5351, -1.9165) (-10.4315, -1.8543) (-10.3258, -1.7957) (-10.2182, -1.7406) (-10.1445, -1.708) (-10.1077, -1.6917) knots -0.096663 -0.096663 -0.096663 -0.096663 -0.072499 -0.060415 -0.048332 -0.036249 -0.024166 -0.012083 0 0 0 0 projected
  arc A75 (-10.161, -1.3341) -> (-10.1077, -1.6917) centre (0, 0) ccw projected
  spline S75 degree 3 poles (-10.161, -1.3341) (-10.201, -1.3292) (-10.281, -1.3196) (-10.4, -1.2983) (-10.5182, -1.2731) (-10.6355, -1.2439) (-10.7518, -1.2111) (-10.9057, -1.1633) (-11.019, -1.1212) (-11.0945, -1.0932) knots -0.096663 -0.096663 -0.096663 -0.096663 -0.084581 -0.072498 -0.060415 -0.048331 -0.036248 -0.024165 0 0 0 0 projected
  arc A76 (-11.1129, -0.8865) -> (-11.0945, -1.0932) centre (0, 0) ccw projected
  spline S76 degree 3 poles (-11.1129, -0.8865) (-11.0435, -0.8456) (-10.9394, -0.7842) (-10.7965, -0.7099) (-10.6878, -0.657) (-10.5775, -0.6075) (-10.4657, -0.5618) (-10.3523, -0.5199) (-10.2753, -0.4962) (-10.2368, -0.4843) knots -0.096663 -0.096663 -0.096663 -0.096663 -0.072499 -0.060415 -0.048332 -0.036249 -0.024166 -0.012083 0 0 0 0 projected
  arc A77 (-10.2475, -0.1229) -> (-10.2368, -0.4843) centre (0, 0) ccw projected
  spline S77 degree 3 poles (-10.2475, -0.1229) (-10.2866, -0.1134) (-10.3649, -0.0943) (-10.4806, -0.0592) (-10.595, -0.0202) (-10.708, 0.0227) (-10.8196, 0.069) (-10.9667, 0.1348) (-11.0742, 0.1899) (-11.1459, 0.2266) knots -0.096663 -0.096663 -0.096663 -0.096663 -0.084581 -0.072498 -0.060415 -0.048331 -0.036248 -0.024165 0 0 0 0 projected
  arc A78 (-11.1398, 0.434) -> (-11.1459, 0.2266) centre (0, 0) ccw projected
  spline S78 degree 3 poles (-11.1398, 0.434) (-11.066, 0.4665) (-10.9554, 0.5152) (-10.8046, 0.572) (-10.6905, 0.6117) (-10.5752, 0.6478) (-10.4587, 0.6799) (-10.3411, 0.7082) (-10.2619, 0.7226) (-10.2222, 0.7298) knots -0.096663 -0.096663 -0.096663 -0.096663 -0.072499 -0.060415 -0.048332 -0.036249 -0.024166 -0.012083 0 0 0 0 projected
  arc A79 (-10.1901, 1.0899) -> (-10.2222, 0.7298) centre (0, 0) ccw projected
  spline S79 degree 3 poles (-10.1901, 1.0899) (-10.2279, 1.104) (-10.3033, 1.1322) (-10.414, 1.1808) (-10.523, 1.2331) (-10.6301, 1.289) (-10.7354, 1.3482) (-10.8738, 1.4309) (-10.9741, 1.4983) (-11.0409, 1.5433) knots -0.096663 -0.096663 -0.096663 -0.096663 -0.084581 -0.072498 -0.060415 -0.048331 -0.036248 -0.024165 0 0 0 0 projected
  arc A80 (-11.0103, 1.7485) -> (-11.0409, 1.5433) centre (0, 0) ccw projected
  spline S80 degree 3 poles (-11.0103, 1.7485) (-10.9332, 1.772) (-10.8176, 1.8073) (-10.6611, 1.8459) (-10.5431, 1.8718) (-10.4243, 1.894) (-10.3048, 1.9121) (-10.1848, 1.9263) (-10.1044, 1.9312) (-10.0642, 1.9337) knots -0.096663 -0.096663 -0.096663 -0.096663 -0.072499 -0.060415 -0.048332 -0.036249 -0.024166 -0.012083 0 0 0 0 projected
  arc A81 (-9.9897, 2.2875) -> (-10.0642, 1.9337) centre (0, 0) ccw projected
  spline S81 degree 3 poles (-9.9897, 2.2875) (-10.0255, 2.306) (-10.0971, 2.3429) (-10.2013, 2.4042) (-10.3033, 2.469) (-10.403, 2.5372) (-10.5006, 2.6085) (-10.6282, 2.7069) (-10.7198, 2.7858) (-10.7809, 2.8383) knots -0.096663 -0.096663 -0.096663 -0.096663 -0.084581 -0.072498 -0.060415 -0.048331 -0.036248 -0.024165 0 0 0 0 projected
  arc A82 (-10.7262, 3.0385) -> (-10.7809, 2.8383) centre (0, 0) ccw projected
  spline S82 degree 3 poles (-10.7262, 3.0385) (-10.6469, 3.0527) (-10.5279, 3.074) (-10.368, 3.0939) (-10.2477, 3.1056) (-10.1271, 3.1136) (-10.0063, 3.1175) (-9.8855, 3.1174) (-9.805, 3.1127) (-9.7648, 3.1104) knots -0.096663 -0.096663 -0.096663 -0.096663 -0.072499 -0.060415 -0.048332 -0.036249 -0.024166 -0.012083 0 0 0 0 projected
  arc A83 (-9.649, 3.4529) -> (-9.7648, 3.1104) centre (0, 0) ccw projected
  spline S83 degree 3 poles (-9.649, 3.4529) (-9.6824, 3.4755) (-9.7491, 3.5206) (-9.8453, 3.5939) (-9.939, 3.6703) (-10.0299, 3.7498) (-10.1184, 3.8321) (-10.2335, 3.9449) (-10.3151, 4.0341) (-10.3695, 4.0935) knots -0.096663 -0.096663 -0.096663 -0.096663 -0.084581 -0.072498 -0.060415 -0.048331 -0.036248 -0.024165 0 0 0 0 projected
  arc A84 (-10.2915, 4.2858) -> (-10.3695, 4.0935) centre (0, 0) ccw projected
  spline S84 degree 3 poles (-10.2915, 4.2858) (-10.2111, 4.2905) (-10.0904, 4.2976) (-9.9293, 4.2984) (-9.8085, 4.2959) (-9.6878, 4.2896) (-9.5674, 4.2791) (-9.4474, 4.2647) (-9.3681, 4.2506) (-9.3284, 4.2435) knots -0.096663 -0.096663 -0.096663 -0.096663 -0.072499 -0.060415 -0.048332 -0.036249 -0.024166 -0.012083 0 0 0 0 projected
  arc A85 (-9.1729, 4.5699) -> (-9.3284, 4.2435) centre (0, 0) ccw projected
  spline S85 degree 3 poles (-9.1729, 4.5699) (-9.2034, 4.5963) (-9.2643, 4.649) (-9.3511, 4.7331) (-9.4351, 4.82) (-9.516, 4.9097) (-9.5942, 5.002) (-9.6951, 5.1276) (-9.7656, 5.2258) (-9.8126, 5.2912) knots -0.096663 -0.096663 -0.096663 -0.096663 -0.084581 -0.072498 -0.060415 -0.048331 -0.036248 -0.024165 0 0 0 0 projected
  arc A86 (-9.7124, 5.4729) -> (-9.8126, 5.2912) centre (0, 0) ccw projected
  spline S86 degree 3 poles (-9.7124, 5.4729) (-9.632, 5.4681) (-9.5113, 5.4609) (-9.3512, 5.4426) (-9.2316, 5.4258) (-9.1125, 5.4052) (-8.9941, 5.3806) (-8.8767, 5.3521) (-8.7996, 5.3287) (-8.761, 5.317) knots -0.096663 -0.096663 -0.096663 -0.096663 -0.072499 -0.060415 -0.048332 -0.036249 -0.024166 -0.012083 0 0 0 0 projected
  arc A87 (-8.568, 5.6228) -> (-8.761, 5.317) centre (0, 0) ccw projected
  spline S87 degree 3 poles (-8.568, 5.6228) (-8.5952, 5.6525) (-8.6494, 5.7121) (-8.7257, 5.8059) (-8.7988, 5.9021) (-8.8686, 6.0008) (-8.9352, 6.1016) (-9.0206, 6.2383) (-9.079, 6.3441) (-9.1179, 6.4146) knots -0.096663 -0.096663 -0.096663 -0.096663 -0.084581 -0.072498 -0.060415 -0.048331 -0.036248 -0.024165 0 0 0 0 projected
  arc A88 (-8.9969, 6.5832) -> (-9.1179, 6.4146) centre (0, 0) ccw projected
  spline S88 degree 3 poles (-8.9969, 6.5832) (-8.9176, 6.5689) (-8.7987, 6.5475) (-8.6419, 6.5104) (-8.525, 6.4796) (-8.4092, 6.4451) (-8.2946, 6.4066) (-8.1814, 6.3644) (-8.1076, 6.3321) (-8.0707, 6.3159) knots -0.096663 -0.096663 -0.096663 -0.096663 -0.072499 -0.060415 -0.048332 -0.036249 -0.024166 -0.012083 0 0 0 0 projected
  arc A89 (-7.8429, 6.5967) -> (-8.0707, 6.3159) centre (0, 0) ccw projected
  spline S89 degree 3 poles (-7.8429, 6.5967) (-7.8663, 6.6294) (-7.9131, 6.695) (-7.9778, 6.7971) (-8.039, 6.9013) (-8.0966, 7.0076) (-8.1509, 7.1155) (-8.2194, 7.2614) (-8.2649, 7.3734) (-8.2952, 7.448) knots -0.096663 -0.096663 -0.096663 -0.096663 -0.084581 -0.072498 -0.060415 -0.048331 -0.036248 -0.024165 0 0 0 0 projected
  arc A90 (-8.1552, 7.6011) -> (-8.2952, 7.448) centre (0, 0) ccw projected
  spline S90 degree 3 poles (-8.1552, 7.6011) (-8.0781, 7.5775) (-7.9625, 7.5422) (-7.8112, 7.4868) (-7.6988, 7.4424) (-7.5879, 7.3944) (-7.4787, 7.3427) (-7.3712, 7.2874) (-7.3017, 7.2465) (-7.267, 7.2261) knots -0.096663 -0.096663 -0.096663 -0.096663 -0.072499 -0.060415 -0.048332 -0.036249 -0.024166 -0.012083 0 0 0 0 projected
  arc A91 (-7.0076, 7.478) -> (-7.267, 7.2261) centre (0, 0) ccw projected
  spline S91 degree 3 poles (-7.0076, 7.478) (-7.027, 7.5133) (-7.0657, 7.5839) (-7.1179, 7.693) (-7.1663, 7.8037) (-7.2109, 7.916) (-7.2521, 8.0296) (-7.3029, 8.1825) (-7.3348, 8.2991) (-7.3561, 8.3768) knots -0.096663 -0.096663 -0.096663 -0.096663 -0.084581 -0.072498 -0.060415 -0.048331 -0.036248 -0.024165 0 0 0 0 projected
  arc A92 (-7.1989, 8.5123) -> (-7.3561, 8.3768) centre (0, 0) ccw projected
  spline S92 degree 3 poles (-7.1989, 8.5123) (-7.1252, 8.4798) (-7.0146, 8.431) (-6.8709, 8.3581) (-6.7646, 8.3007) (-6.6601, 8.24) (-6.5577, 8.1757) (-6.4576, 8.108) (-6.3934, 8.0593) (-6.3614, 8.0349) knots -0.096663 -0.096663 -0.096663 -0.096663 -0.072499 -0.060415 -0.048332 -0.036249 -0.024166 -0.012083 0 0 0 0 projected
  arc A93 (-6.074, 8.2543) -> (-6.3614, 8.0349) centre (0, 0) ccw projected
  spline S93 degree 3 poles (-6.074, 8.2543) (-6.089, 8.2916) (-6.1192, 8.3664) (-6.158, 8.4808) (-6.193, 8.5965) (-6.2241, 8.7133) (-6.2515, 8.831) (-6.2839, 8.9889) (-6.3018, 9.1084) (-6.3137, 9.1881) knots -0.096663 -0.096663 -0.096663 -0.096663 -0.084581 -0.072498 -0.060415 -0.048331 -0.036248 -0.024165 0 0 0 0 projected
  arc A94 (-6.1416, 9.304) -> (-6.3137, 9.1881) centre (0, 0) ccw projected
  spline S94 degree 3 poles (-6.1416, 9.304) (-6.0723, 9.263) (-5.9682, 9.2015) (-5.8341, 9.1121) (-5.7353, 9.0425) (-5.6388, 8.9698) (-5.5447, 8.8939) (-5.4533, 8.8149) (-5.3954, 8.7589) (-5.3664, 8.7309) knots -0.096663 -0.096663 -0.096663 -0.096663 -0.072499 -0.060415 -0.048332 -0.036249 -0.024166 -0.012083 0 0 0 0 projected
  arc A95 (-5.0551, 8.9147) -> (-5.3664, 8.7309) centre (0, 0) ccw projected
  spline S95 degree 3 poles (-5.0551, 8.9147) (-5.0656, 8.9536) (-5.0867, 9.0314) (-5.1117, 9.1496) (-5.1328, 9.2686) (-5.1498, 9.3883) (-5.1631, 9.5084) (-5.1766, 9.669) (-5.1803, 9.7898) (-5.1827, 9.8703) knots -0.096663 -0.096663 -0.096663 -0.096663 -0.084581 -0.072498 -0.060415 -0.048331 -0.036248 -0.024165 0 0 0 0 projected
  arc A96 (-4.9981, 9.9651) -> (-5.1827, 9.8703) centre (0, 0) ccw projected
  spline S96 degree 3 poles (-4.9981, 9.9651) (-4.9341, 9.9161) (-4.838, 9.8428) (-4.7154, 9.7382) (-4.6256, 9.6574) (-4.5383, 9.5738) (-4.4539, 9.4873) (-4.3724, 9.398) (-4.3215, 9.3355) (-4.2961, 9.3043) knots -0.096663 -0.096663 -0.096663 -0.096663 -0.072499 -0.060415 -0.048332 -0.036249 -0.024166 -0.012083 0 0 0 0 projected
  arc A97 (-3.9652, 9.45) -> (-4.2961, 9.3043) centre (0, 0) ccw projected
  spline S97 degree 3 poles (-3.9652, 9.45) (-3.9711, 9.4899) (-3.9828, 9.5696) (-3.9937, 9.69) (-4.0006, 9.8106) (-4.0033, 9.9315) (-4.0023, 10.0523) (-3.9967, 10.2134) (-3.986, 10.3337) (-3.9789, 10.414) knots -0.096663 -0.096663 -0.096663 -0.096663 -0.084581 -0.072498 -0.060415 -0.048331 -0.036248 -0.024165 0 0 0 0 projected
  arc A98 (-3.7844, 10.4863) -> (-3.9789, 10.414) centre (0, 0) ccw projected
  spline S98 degree 3 poles (-3.7844, 10.4863) (-3.7266, 10.4301) (-3.64, 10.3459) (-3.5306, 10.2275) (-3.4509, 10.1367) (-3.3741, 10.0433) (-3.3006, 9.9475) (-3.2302, 9.8492) (-3.1871, 9.7811) (-3.1655, 9.7471) knots -0.096663 -0.096663 -0.096663 -0.096663 -0.072499 -0.060415 -0.048332 -0.036249 -0.024166 -0.012083 0 0 0 0 projected
  arc A99 (-2.8197, 9.8527) -> (-3.1655, 9.7471) centre (0, 0) ccw projected
  spline S99 degree 3 poles (-2.8197, 9.8527) (-2.8208, 9.893) (-2.8231, 9.9735) (-2.8196, 10.0943) (-2.8122, 10.215) (-2.8006, 10.3353) (-2.7853, 10.4551) (-2.7607, 10.6144) (-2.7359, 10.7327) (-2.7193, 10.8115) knots -0.096663 -0.096663 -0.096663 -0.096663 -0.084581 -0.072498 -0.060415 -0.048331 -0.036248 -0.024165 0 0 0 0 projected
  arc A100 (-2.5176, 10.8602) -> (-2.7193, 10.8115) centre (0, 0) ccw projected
  spline S100 degree 3 poles (-2.5176, 10.8602) (-2.4669, 10.7977) (-2.3908, 10.7038) (-2.2962, 10.5733) (-2.2278, 10.4737) (-2.1626, 10.3719) (-2.1009, 10.268) (-2.0426, 10.1621) (-2.0079, 10.0894) (-1.9905, 10.0531) knots -0.096663 -0.096663 -0.096663 -0.096663 -0.072499 -0.060415 -0.048332 -0.036249 -0.024166 -0.012083 0 0 0 0 projected
  arc A101 (-1.6346, 10.117) -> (-1.9905, 10.0531) centre (0, 0) ccw projected
  spline S101 degree 3 poles (-1.6346, 10.117) (-1.631, 10.1572) (-1.6236, 10.2374) (-1.6059, 10.357) (-1.5843, 10.4759) (-1.5586, 10.5939) (-1.5292, 10.7112) (-1.4859, 10.8664) (-1.4473, 10.9809) (-1.4215, 11.0572) knots -0.096663 -0.096663 -0.096663 -0.096663 -0.084581 -0.072498 -0.060415 -0.048331 -0.036248 -0.024165 0 0 0 0 projected
  arc A102 (-1.2155, 11.0818) -> (-1.4215, 11.0572) centre (0, 0) ccw projected
  spline S102 degree 3 poles (-1.2155, 11.0818) (-1.1725, 11.0136) (-1.108, 10.9114) (-1.0295, 10.7707) (-0.9734, 10.6636) (-0.9207, 10.5549) (-0.8717, 10.4444) (-0.8264, 10.3323) (-0.8005, 10.2561) (-0.7875, 10.2179) knots -0.096663 -0.096663 -0.096663 -0.096663 -0.072499 -0.060415 -0.048332 -0.036249 -0.024166 -0.012083 0 0 0 0 projected
  arc A103 (-0.4266, 10.2394) -> (-0.7875, 10.2179) centre (0, 0) ccw projected
  spline S103 degree 3 poles (-0.4266, 10.2394) (-0.4182, 10.2788) (-0.4014, 10.3576) (-0.3697, 10.4742) (-0.3341, 10.5897) (-0.2946, 10.7039) (-0.2516, 10.8168) (-0.1903, 10.9659) (-0.1384, 11.075) (-0.1037, 11.1478) knots -0.096663 -0.096663 -0.096663 -0.096663 -0.084581 -0.072498 -0.060415 -0.048331 -0.036248 -0.024165 0 0 0 0 projected
  arc A104 (0.1037, 11.1478) -> (-0.1037, 11.1478) centre (0, 0) ccw projected
  spline S104 degree 3 poles (0.1037, 11.1478) (0.1384, 11.075) (0.1903, 10.9659) (0.2516, 10.8168) (0.2946, 10.7039) (0.3341, 10.5897) (0.3697, 10.4742) (0.4014, 10.3576) (0.4182, 10.2788) (0.4266, 10.2394) knots -0.096663 -0.096663 -0.096663 -0.096663 -0.072499 -0.060415 -0.048332 -0.036249 -0.024166 -0.012083 0 0 0 0 projected
  arc A105 (0.7875, 10.2179) -> (0.4266, 10.2394) centre (0, 0) ccw projected
  spline S105 degree 3 poles (0.7875, 10.2179) (0.8005, 10.2561) (0.8264, 10.3323) (0.8717, 10.4444) (0.9207, 10.5549) (0.9734, 10.6636) (1.0295, 10.7707) (1.108, 10.9114) (1.1725, 11.0136) (1.2155, 11.0818) knots -0.096663 -0.096663 -0.096663 -0.096663 -0.084581 -0.072498 -0.060415 -0.048331 -0.036248 -0.024165 0 0 0 0 projected
  arc A106 (1.4215, 11.0572) -> (1.2155, 11.0818) centre (0, 0) ccw projected
  circle A107 centre (0, 0) radius 12.0482 projected
  dimension "d0" = 1
  constraints: 1 centre point, 1 coincident
  measures "d0" radial gap between concentric circles of A107 A0
extrude "Extrusion1" add sketch "Sketch1" against normal blind 2 contours A0
sketch "Sketch2" plane through (0, 0, 0) normal (0, 0, 1) x (1, 0, 0)
  circle A0 centre (0, 0) radius 13.0482 projected
  circle A1 centre (0, 0) radius 13.0482
  circle A2 centre (0, 0) radius 11.0482
  dimension "d3" = 2
  constraints: 2 centre point, 2 coincident, 1 concentric
  measures "d3" radial gap between concentric circles of A1 A2
extrude "Extrusion2" add sketch "Sketch2" along normal blind 2
body "Solid1"
